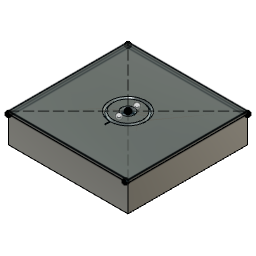
TopCover v3 (Autodesk Fusion 360 design; units mm, degrees)
Autodesk Fusion 360 part; units mm, degrees
sketch "Sketch1" plane through (0, 0, 0) normal (0, 0, 1) x (1, 0, 0)
cylinder "CylinderPrimitive1" add diameter 42 height 2 placed x (1, 0, 0) y (0, 1, 0) z (0, 0, 1) at (0, 0, 0) makes body 1
cylinder "CylinderPrimitive2" add diameter 42 height 15 placed x (1, 0, 0) y (0, 1, 0) z (0, 0, 1) at (0, 0, 2) bodies 1
hole "Hole1" at (0, 0, 17) direction (0, 0, -1) diameter 40.35 depth 15 tip angle 180 bodies 1
cylinder "CylinderPrimitive3" add diameter 36.6 height 20 placed x (1, 0, 0) y (0, 1, 0) z (0, 0, 1) at (0, 0, 0) bodies 1
hole "Hole2" at (0, 0, 20) direction (0, 0, -1) diameter 34 depth 20 tip angle 180 bodies 1
copy_body "Body->Comp1" bodies 1 removing the originals makes body 2 in component "Component"
sketch "Sketch1 (2)" plane through (0, 0, 0) normal (0, 0, 1) x (1, 0, 0) in component "TopCover"
  line L0 (-73.5, -73.5) -> (73.5, -73.5)
  line L1 (73.5, -73.5) -> (73.5, 73.5)
  line L2 (73.5, 73.5) -> (-73.5, 73.5)
  line L3 (-73.5, 73.5) -> (-73.5, -73.5)
  line L4 (-73.5, -73.5) -> (73.5, 73.5) construction
  line L5 (73.5, -73.5) -> (-73.5, 73.5) construction
  dimension "d13" = 147
  dimension "d14" = 147
  constraint horizontal L0
  constraint perpendicular L0 L1
  constraint parallel L0 L2
  constraint parallel L1 L3
  constraint coincident L4 origin
  constraint coincident L5 origin
  measures "d13" distance of L1.end L2.end
  measures "d14" distance of L0.end L1.end
extrude "Extrude1" add sketch "Sketch1 (2)" against normal blind 3 separate body makes body 3 in component "TopCover"
sketch "Sketch2" plane through (0, 0, -3) normal (0, 0, -1) x (1, 0, 0) in component "TopCover"
  line L0 (-73.5, 73.5) -> (-73.5, -73.5)
  line L1 (-73.5, -73.5) -> (73.5, -73.5)
  line L2 (73.5, -73.5) -> (73.5, 73.5)
  line L3 (73.5, 73.5) -> (-73.5, 73.5)
  line L4 (73.5, -73.5) -> (70.5, -73.5)
  line L5 (70.5, -73.5) -> (70.5, 73.5)
  line L6 (70.5, 73.5) -> (73.5, 73.5)
  line L7 (73.5, 73.5) -> (73.5, -73.5)
  line L8 (-73.5, -73.5) -> (-70.5, -73.5)
  line L9 (-70.5, -73.5) -> (-70.5, 73.5)
  line L10 (-70.5, 73.5) -> (-73.5, 73.5)
  line L11 (-73.5, 73.5) -> (-73.5, -73.5)
  line L12 (-70.5, 73.5) -> (70.5, 73.5)
  line L13 (70.5, 73.5) -> (70.5, 70.5)
  line L14 (70.5, 70.5) -> (-70.5, 70.5)
  line L15 (-70.5, 70.5) -> (-70.5, 73.5)
  line L16 (-70.5, -73.5) -> (70.5, -73.5)
  line L17 (70.5, -73.5) -> (70.5, -70.5)
  line L18 (70.5, -70.5) -> (-70.5, -70.5)
  line L19 (-70.5, -70.5) -> (-70.5, -73.5)
  dimension "d17" = 3
  dimension "d18" = 3
  dimension "d23" = 3
  dimension "d24" = 3
  constraint horizontal L4
  constraint vertical L5
  constraint horizontal L6
  constraint vertical L7
  constraint coincident L1.end L2.start
  constraint horizontal L8
  constraint vertical L9
  constraint horizontal L10
  constraint vertical L11
  constraint coincident L0.end L1.start
  constraint coincident L0.start L3.end
  constraint coincident L3 L5.end
  constraint horizontal L12
  constraint vertical L13
  constraint horizontal L14
  constraint vertical L15
  constraint horizontal L16
  constraint vertical L17
  constraint horizontal L18
  constraint vertical L19
  constraint coincident L5 L17.end
  measures "d17" distance of L1.end L4.end
  measures "d18" distance of L0.end L8.end
  measures "d23" distance of L9.end L14.end
  measures "d24" distance of L8.end L18.end
extrude "Extrude2" add sketch "Sketch2" along normal blind 33 contours L0 L1 L3 L8 L9 L10 L11 L15 L19 bodies 3 in component "TopCover"
extrude "Extrude3" add sketch "Sketch2" along normal blind 33 contours L1 L2 L3 L4 L5 L6 L7 L13 L17 bodies 3 in component "TopCover"
extrude "Extrude4" add sketch "Sketch2" along normal blind 33 contours L3 L5 L9 L12 L13 L14 L15 bodies 3 in component "TopCover"
extrude "Extrude5" add sketch "Sketch2" along normal blind 33 contours L1 L5 L9 L16 L17 L18 L19 bodies 3 in component "TopCover"
sketch "Sketch3" plane through (0, 0, -3) normal (0, 0, -1) x (1, 0, 0) in component "TopCover"
  arc A0 (70.5, 70.5) -> (70.5, -70.5) centre (111.6111, 0) ccw
  arc A1 (70.5, -70.5) -> (-70.5, -70.5) centre (0, -112.7814) ccw
  arc A2 (-70.5, -70.5) -> (-70.5, 70.5) centre (-108.5568, 0) ccw
  arc A3 (-70.5, 70.5) -> (70.5, 70.5) centre (0, 111.6111) ccw
  line L0 (-52.8048, 57.5351) -> (-28.4354, 35.114)
  line L1 (53.8282, 57.6325) -> (28.4354, 35.114)
  line L2 (57.9865, 54.1834) -> (35.714, 30)
  line L3 (57.4361, -53.9676) -> (35.714, -30)
  line L4 (54.138, -57.9415) -> (30.4205, -36.4102)
  line L5 (-55.1072, -59.6801) -> (-28.1638, -35.5495)
  line L6 (-56.0257, -52.6225) -> (-34.3817, -30.2758)
  line L7 (-55.8235, 52.0787) -> (-34.2733, 30.0088)
  point P0 (-70.5, 70.5)
  point P1 (70.5, 70.5)
  point P2 (70.5, -70.5)
  point P3 (-70.5, -70.5)
  constraint coincident A0.start A3.end
  constraint coincident P2 A0.end
  constraint coincident P3 A1.end
  constraint coincident P0 A2.end
  constraint coincident P1 A0.start
  constraint coincident A2 L0.start
  constraint coincident A3 L0.end
  constraint coincident A0 L1.start
  constraint coincident A3 L1.end
  constraint coincident A3 L2.start
  constraint coincident A0 L2.end
  constraint coincident A1 L3.start
  constraint coincident A0 L3.end
  constraint coincident A0 L4.start
  constraint coincident A1 L4.end
  constraint coincident A2 L5.start
  constraint coincident A1 L5.end
  constraint tangent A2 L5
  constraint coincident A1 L6.start
  constraint coincident A2 L6.end
  constraint coincident A3 L7.start
  constraint coincident A2 L7.end
extrude "Extrude6" add sketch "Sketch3" along normal blind 1 separate body makes body 4 in component "TopCover"
cylinder "CylinderPrimitive1'" add diameter 43 height 16 placed x (0, 1, 0) y (1, 0, 0) z (0, 0, -1) at (0, 0, -3) bodies 4 3 in component "TopCover"
hole "Hole3" at (0, 0, 0) direction (0, 0, -1) diameter 40.35 depth 13 tip angle 180 countersink diameter 44.385 countersink angle 90 bodies 4 in component "TopCover"
cylinder "CylinderPrimitive2'" add diameter 36.6 height -13 placed x (1, 0, 0) y (0, 1, 0) z (0, 0, 1) at (0, 0, 0) separate body makes body 5 in component "TopCover"
hole "Hole4" at (0, 0, -19) direction (0, 0, 1) diameter 30 depth 13 tip angle 180 bodies 4 5 in component "TopCover"
sketch "Sketch4" plane through (0, 0, -3) normal (0, 0, -1) x (1, 0, 0) in component "TopCover"
  line L0 (-55.5, 70.5) -> (-47.5, 70.5)
  line L1 (-47.5, 70.5) -> (-47.5, 66.5)
  line L2 (-47.5, 66.5) -> (-55.5, 66.5)
  line L3 (-55.5, 66.5) -> (-55.5, 70.5)
  line L4 (70.5, 70.5) -> (-70.5, 70.5)
  line L5 (55.5, 70.5) -> (55.5, 66.5)
  line L6 (47.5, 70.5) -> (55.5, 70.5)
  line L7 (47.5, 66.5) -> (47.5, 70.5)
  line L8 (55.5, 66.5) -> (47.5, 66.5)
  line L9 (-55.5, -70.5) -> (-47.5, -70.5)
  line L10 (-47.5, -70.5) -> (-47.5, -66.5)
  line L11 (-47.5, -66.5) -> (-55.5, -66.5)
  line L12 (-55.5, -66.5) -> (-55.5, -70.5)
  line L13 (70.5, -70.5) -> (-70.5, -70.5)
  line L14 (47.5, -70.5) -> (55.5, -70.5)
  line L15 (55.5, -70.5) -> (55.5, -66.5)
  line L16 (55.5, -66.5) -> (47.5, -66.5)
  line L17 (47.5, -66.5) -> (47.5, -70.5)
  line L18 (-70.5, 55.5) -> (-66.5, 55.5)
  line L19 (-66.5, 55.5) -> (-66.5, 47.5)
  line L20 (-66.5, 47.5) -> (-70.5, 47.5)
  line L21 (-70.5, 47.5) -> (-70.5, 55.5)
  line L22 (-70.5, -73.5) -> (-70.5, 73.5)
  line L23 (-70.5, -47.5) -> (-66.5, -47.5)
  line L24 (-66.5, -47.5) -> (-66.5, -55.5)
  line L25 (-66.5, -55.5) -> (-70.5, -55.5)
  line L26 (-70.5, -55.5) -> (-70.5, -47.5)
  line L27 (70.5, 55.5) -> (66.5, 55.5)
  line L28 (66.5, 55.5) -> (66.5, 47.5)
  line L29 (66.5, 47.5) -> (70.5, 47.5)
  line L30 (70.5, 47.5) -> (70.5, 55.5)
  line L31 (70.5, -73.5) -> (70.5, 73.5)
  line L32 (70.5, -47.5) -> (66.5, -47.5)
  line L33 (66.5, -47.5) -> (66.5, -55.5)
  line L34 (66.5, -55.5) -> (70.5, -55.5)
  line L35 (70.5, -55.5) -> (70.5, -47.5)
  dimension "d31" = 8
  dimension "d32" = 4
  dimension "d33" = 8
  dimension "d34" = 4
  dimension "d35" = 15
  dimension "d36" = 15
  dimension "d37" = 8
  dimension "d38" = 4
  dimension "d39" = 8
  dimension "d40" = 4
  dimension "d41" = 4
  dimension "d42" = 8
  dimension "d43" = 4
  dimension "d44" = 8
  dimension "d45" = 4
  dimension "d46" = 8
  dimension "d47" = 4
  dimension "d48" = 8
  dimension "d49" = 15
  dimension "d50" = 15
  dimension "d51" = 15
  dimension "d52" = 15
  dimension "d53" = 15
  dimension "d54" = 15
  constraint horizontal L0
  constraint vertical L1
  constraint horizontal L2
  constraint vertical L3
  constraint coincident L0.start L4
  constraint horizontal L6
  constraint vertical L5
  constraint horizontal L8
  constraint vertical L7
  constraint horizontal L9
  constraint vertical L10
  constraint horizontal L11
  constraint vertical L12
  constraint coincident L9.start L13
  constraint horizontal L14
  constraint vertical L15
  constraint horizontal L16
  constraint vertical L17
  constraint coincident L13 L14.start
  constraint horizontal L18
  constraint vertical L19
  constraint horizontal L20
  constraint vertical L21
  constraint coincident L18.start L22
  constraint horizontal L23
  constraint vertical L24
  constraint horizontal L25
  constraint vertical L26
  constraint coincident L22 L23.start
  constraint horizontal L27
  constraint vertical L28
  constraint horizontal L29
  constraint vertical L30
  constraint coincident L27.start L31
  constraint horizontal L32
  constraint vertical L33
  constraint horizontal L34
  constraint vertical L35
  constraint coincident L31 L32.start
  measures "d31" distance of L0.start L0.end
  measures "d32" distance of L0.start L2.end
  measures "d33" distance of L6.start L5.start
  measures "d34" distance of L7.start L6.start
  measures "d35" distance of L0.start L4.end
  measures "d36" distance of L4.start L5.start
  measures "d37" distance of L9.start L9.end
  measures "d38" distance of L9.start L11.end
  measures "d39" distance of L14.start L14.end
  measures "d40" distance of L14.start L16.end
  measures "d41" distance of L18.start L18.end
  measures "d42" distance of L18.start L20.end
  measures "d43" distance of L23.start L23.end
  measures "d44" distance of L23.start L25.end
  measures "d45" distance of L27.start L27.end
  measures "d46" distance of L27.start L29.end
  measures "d47" distance of L32.start L32.end
  measures "d48" distance of L32.start L34.end
  measures "d49" distance of L4.start L27.start
  measures "d50" distance of L13.start L34.end
  measures "d51" distance of L13.start L14.end
  measures "d52" distance of L9.start L13.end
  measures "d53" distance of L13.end L25.end
  measures "d54" distance of L4.end L18.start
extrude "Extrude7" add sketch "Sketch4" along normal blind 18 contours L0 L1 L2 L3 L4 | L4 L5 L6 L7 L8 | L18 L19 L20 L21 L22 | L22 L23 L24 L25 L26 | L27 L28 L29 L30 L31 | L31 L32 L33 L34 L35 | L9 L10 L11 L12 L13 | L13 L14 L15 L16 L17 bodies 4 in component "TopCover"
hole "Hole1'" at (0, 0, 0) direction (0, 0, -1) diameter 15.5 depth 10 tip angle 180 bodies 5 in component "TopCover"
sketch "Sketch5" plane through (0, 0, 0) normal (0, 0, 1) x (1, 0, 0) in component "TopCover"
  point P0 (0, -11)
  point P1 (0, 11)
  dimension "d60" = 11
  dimension "d61" = 11
  measures "d60" distance of origin P0
  measures "d61" distance of origin P1
hole "Hole2'" at (0, 11, 0) at (0, -11, 0) direction (0, 0, -1) diameter 3 depth 6 tip angle 180 countersink diameter 4 countersink angle 90 bodies 5 in component "TopCover"
sketch "Sketch9" plane through (0, 0, 0) normal (0, 0, 1) x (1, 0, 0) in component "TopCover"
  line L0 (0.5, -22) -> (-0.5, -22)
  line L1 (-0.5, -22) -> (-0.5, -28)
  line L2 (-0.5, -28) -> (0.5, -28)
  line L3 (0.5, -28) -> (0.5, -22)
  line L4 (0.5, -22) -> (-0.5, -28) construction
  line L5 (-0.5, -22) -> (0.5, -28) construction
  point P0 (0, -25)
  dimension "d79" = 1
  dimension "d80" = 6
  constraint horizontal L0
  constraint perpendicular L0 L1
  constraint parallel L0 L2
  constraint parallel L1 L3
  constraint coincident L4 P0
  constraint coincident L5 P0
  measures "d79" distance of L1.end L2.end
  measures "d80" distance of L0.end L1.end
extrude "Extrude8" cut sketch "Sketch9" against normal blind 1 bodies 4 in component "TopCover"
component "TopCover" placed x (1, 0, 0) y (0, 1, 0) z (0, 0, 1) at (0, 0, 0)
component "Component" placed x (1, 0, 0) y (0, 1, 0) z (0, 0, 1) at (0, 0, 0)
